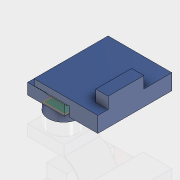
# Autodesk Inventor part: ЛЦМК0000002.00.00.00.00.04
Saved by Autodesk Inventor 2021.2 (Build 252289000, 289)
## iProperties
Created: 2025-10-23
Part Number: ЛЦМК0000002.00.00.00.00.04
Material: Типовые
Document SubType Name: Modeling
Designer: Захаров
Density: 1 g/cm^3
Appearance: С вкраплениями — сатинированная — синяя
Author: Захаров
Autodesk Inventor part; units mm, degrees
ref_plane "YZ Plane" through (0, 0, 0) normal (1, 0, 0) x (0, 1, 0)
ref_plane "XZ Plane" through (0, 0, 0) normal (0, 1, 0) x (-1, 0, 0)
ref_plane "РабПлоскость1" through (116.75, -2.8, -7.7) normal (0, -1, 0) x (1, 0, 0)
sketch "Эскиз1" plane through (116.75, -2.8, -7.7) normal (0, -1, 0) x (1, 0, 0)
  line L0 (97, 9) -> (112.5, 9)
  line L1 (112.5, 9) -> (112.5, -9)
  line L2 (112.5, -9) -> (97, -9)
  line L3 (112.5, 2.2) -> (109.5, 2.2)
  line L4 (109.5, 2.2) -> (109.5, -6.5)
  line L5 (112.5, -6.5) -> (112.5, 2.2)
  line L6 (109.5, -6.5) -> (112.5, -6.5)
  line L7 (97, 9) -> (97, -9)
  point P0 (-116.75, 7.7)
  dimension "d9" = 15.5
  dimension "d10" = 3
  dimension "d11" = 8.7
  dimension "d13" = 2.5
  constraints: 16 end point, 3 horizontal, 2 parallel, 2 perpendicular, 1 point on line, 1 vertical
  measures "d9" distance of L1.end L2.end
  measures "d10" distance of L5.start L4.end
  measures "d11" distance of L4.end L3.end
  measures "d13" distance between parallel lines of L2 L6
extrude "Выдавливание1" add sketch "Эскиз1" along normal blind 1.5
sketch "Эскиз5" plane through (116.75, -2.8, -7.7) normal (0, 1, 0) x (1, 0, 0)
  line L0 (112.5, 9) -> (112.5, -9) projected
  line L1 (112.5, 2.2) -> (109.5, 2.2)
  line L2 (109.5, 2.2) -> (109.5, -6.5)
  line L3 (109.5, -6.5) -> (112.5, -6.5)
  line L4 (112.5, -6.5) -> (112.5, 2.2)
  line L5 (112.5, -9) -> (97, -9) projected
  point P0 (-116.75, -7.7)
  point P1 (112.5, -6.5)
  dimension "d14" = 3
  dimension "d15" = 8.7
  dimension "d16" = 2.5
  constraints: 8 end point, 2 parallel, 1 horizontal, 1 perpendicular, 1 point on line
  measures "d14" distance of L3.end L2.end
  measures "d15" distance of L2.end L1.end
  measures "d16" distance between parallel lines of L5 L3
extrude "Выдавливание5" add sketch "Эскиз5" along normal blind 2.8
sketch "Эскиз6" plane through (116.75, -4.3, -7.7) normal (0, -1, 0) x (1, 0, 0)
  line L0 (112.5, 9) -> (97, 9) projected
  line L1 (105.5, 9) -> (112.5, 9)
  line L2 (112.5, 9) -> (112.5, -9)
  line L3 (112.5, -9) -> (105.5, -9)
  line L4 (105.5, -9) -> (105.5, 9)
  point P0 (112.5, 9)
  dimension "d19" = 7
  constraints: 8 end point, 2 parallel, 1 horizontal, 1 perpendicular, 1 point on line
  measures "d19" distance between parallel lines of L2 L4
extrude "Выдавливание6" add sketch "Эскиз6" along normal blind 2.3
sketch "Эскиз7" plane through (116.75, -4.3, -7.7) normal (0, -1, 0) x (1, 0, 0)
  line L0 (97, 5.9073) -> (101.8, 5.9073)
  line L1 (101.8, 5.9073) -> (101.8, -5.6927)
  line L2 (101.8, -5.6927) -> (97, -5.6927)
  line L3 (97, -5.6927) -> (97, 5.9073)
  line L4 (97, 5.9073) -> (101.8, -5.6927) construction
  line L5 (101.8, 5.9073) -> (97, -5.6927) construction
  line L6 (97, 9) -> (97, -9) projected
  point P0 (99.4, 0.1073)
  point P1 (97, 0)
  dimension "d22" = 4.8
  dimension "d23" = 11.6
  constraints: 12 end point, 3 midpoint, 2 parallel, 1 horizontal, 1 perpendicular, 1 point on line
  measures "d22" distance of L1.end L2.end
  measures "d23" distance of L0.end L1.end
extrude "Выдавливание7" add sketch "Эскиз7" along normal blind 3.3
ref_plane "РабПлоскость3" through (116.75, -9.1, -7.7) normal (0, -1, 0) x (1, 0, 0)
sketch "Эскиз8" plane through (116.75, -9.1, -7.7) normal (0, -1, 0) x (1, 0, 0)
  line L0 (99.5911, -4.348) -> (90.6911, -4.348)
  line L1 (90.6911, -4.348) -> (90.6911, 4.252)
  line L2 (90.6911, 4.252) -> (99.5911, 4.252)
  line L3 (99.5911, 4.252) -> (99.5911, -4.348)
  line L4 (99.5911, -4.348) -> (90.6911, 4.252) construction
  line L5 (90.6911, -4.348) -> (99.5911, 4.252) construction
  point P0 (95.1411, -0.048)
  dimension "d27" = 8.9
  dimension "d28" = 8.6
  constraints: 12 end point, 2 midpoint, 2 parallel, 1 horizontal, 1 perpendicular
  measures "d27" distance of L1.end L2.end
  measures "d28" distance of L0.end L1.end
extrude "Выдавливание8" add sketch "Эскиз8" along normal blind 2.7
sketch "Эскиз9" plane through (116.75, -11.8, -7.7) normal (0, -1, 0) x (1, 0, 0)
  line L0 (99.5911, 4.252) -> (90.6911, 4.252) projected
  line L1 (90.6911, 4.252) -> (90.6911, -4.348) projected
  line L2 (90.6911, -4.348) -> (99.5911, -4.348) projected
  line L3 (99.5911, -4.348) -> (99.5911, 4.252) projected
  circle A0 centre (95.1411, -0.048) radius 3.75
  line L4 (99.5911, -4.348) -> (99.5911, 4.252) projected
  line L5 (99.5911, -4.348) -> (90.6911, 4.252) construction
  line L6 (90.6911, 4.252) -> (90.6911, -4.348) projected
  line L7 (99.5911, 4.252) -> (90.6911, 4.252) projected
  line L8 (90.6911, -4.348) -> (99.5911, 4.252) construction
  point P0 (-116.75, 7.7)
  point P1 (95.1411, -0.048)
  dimension "d31" = 7.5
  constraints: 4 end point, 1 centre point, 1 coincident, 1 midpoint
  measures "d31" diameter of A0
extrude "Выдавливание9" add sketch "Эскиз9" along normal blind 3 contours A0
sketch "Эскиз10" plane through (207.4411, -9.1, -3.448) normal (0, 0, 1) x (1, 0, 0)
  line L0 (8.9, 0) -> (8.9, -2.7) projected
  line L1 (8.9, -0.1624) -> (13.3567, 1.2413) construction
  line L2 (13.3567, 1.2413) -> (11.759, 4.6341) construction
  line L3 (11.759, 4.6341) -> (14.8089, 4.6341) construction
  spline S0 degree 3 poles (8.9, -0.1624) (13.3567, 1.2413) (11.759, 4.6341) (14.8089, 4.6341) knots 1 1 1 1 2 2 2 2
  line L4 (14.8089, 4.8) -> (14.8089, 2.5) projected
  line L5 (8.9, 0) -> (8.9, -2.7) projected
  line L6 (8.9, 0) -> (13.3148, 1.3302) construction
  line L7 (13.3148, 1.3302) -> (11.3789, 4.7272) construction
  line L8 (14.8089, 4.8) -> (6.3089, 4.8) projected
  line L9 (11.3789, 4.7272) -> (14.8089, 4.8) construction
  spline S1 degree 3 poles (8.9, 0) (13.3148, 1.3302) (11.3789, 4.7272) (14.8089, 4.8) knots 1 1 1 1 2 2 2 2
  point P0 (-207.4411, 9.1)
  constraints: 4 point on line, 6 other
extrude "Выдавливание10" add sketch "Эскиз10" against normal up to surface (8.6 mm away)
